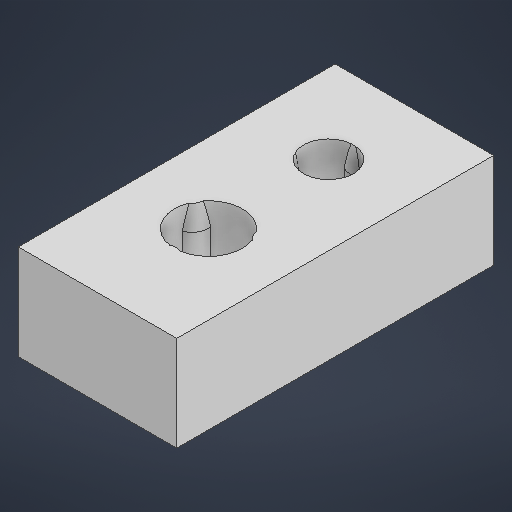
# Autodesk Inventor part: Tolerance_test
Saved by Autodesk Inventor 2025 (Build 290162010, 162A)
## iProperties
Created: 2025-03-10
Part Number: Tolerance_test
Material: Generic
Document SubType Name: Modeling
Designer: tzu98
Density: 1 g/cm^3
Appearance: Default
Author: tzu98
Autodesk Inventor part; units mm, degrees
ref_plane "YZ Plane" through (0, 0, 0) normal (1, 0, 0) x (0, 1, 0)
ref_plane "XZ Plane" through (0, 0, 0) normal (0, 1, 0) x (-1, 0, 0)
ref_plane "XY Plane" through (0, 0, 0) normal (0, 0, 1) x (1, 0, 0)
sketch "Sketch1" plane through (0, 0, 0) normal (0, 0, 1) x (1, 0, 0)
  line L0 (-5, -10) -> (5, -10)
  line L1 (5, -10) -> (5, 10)
  line L2 (5, 10) -> (-5, 10)
  line L3 (-5, 10) -> (-5, -10)
  line L4 (-5, -10) -> (5, 10) construction
  line L5 (5, -10) -> (-5, 10) construction
  circle A0 centre (-10.5904, 5.4479) radius 1.6
  circle A1 centre (-8.5404, 5.4479) radius 0.75
  point P0 (0, 0)
  point P1 (-9.0782, 4.9252)
  point P2 (-9.0782, 5.9707)
  dimension "d0" = 3.2
  dimension "d1" = 2.05
  dimension "d2" = 1.5
  dimension "d29" = 10
  dimension "d30" = 20
  constraints: 12 end point, 2 centre point, 2 midpoint, 2 parallel, 1 horizontal, 1 perpendicular
  measures "d0" diameter of A0
  measures "d1" distance of A1.centre A0.centre
  measures "d2" diameter of A1
  measures "d29" distance between parallel lines of L1 L3
  measures "d30" distance between parallel lines of L2 L0
extrude "Extrusion1" add sketch "Sketch1" along normal blind 6 contours L3 L2 L1 L0
sketch "Sketch2" plane through (0, 0, 6) normal (0, 0, 1) x (1, 0, 0)
  circle A0 centre (0, 4.575) radius 1.575
  line L0 (0, 4.575) -> (0, 6.625)
  circle A1 centre (0, 6.625) radius 0.75
  circle A2 centre (-1.7754, 3.55) radius 0.75
  circle A3 centre (1.7754, 3.55) radius 0.75
  line L1 (0, 0) -> (0, 3)
  circle A4 centre (0, -3) radius 2.15
  line L2 (0, -3) -> (0, -5.8)
  circle A5 centre (0, -5.8) radius 1
  circle A6 centre (2.4249, -1.6) radius 1
  circle A7 centre (-2.4249, -1.6) radius 1
  point P0 (1.0418, 3.3938)
  point P1 (1.5439, 4.2634)
  point P2 (0.5021, 6.0678)
  point P3 (-0.5021, 6.0678)
  point P4 (-1.5439, 4.2634)
  point P5 (-1.0418, 3.3938)
  point P6 (-1.4437, -1.4068)
  point P7 (-2.1016, -2.5463)
  point P8 (-0.6579, -5.0469)
  point P9 (0.6579, -5.0469)
  point P10 (2.1016, -2.5463)
  point P11 (1.4437, -1.4068)
  dimension "d5" = 3.15
  dimension "d6" = 2.05
  dimension "d7" = 1.5
  dimension "d10" = 360
  dimension "d17" = 3
  dimension "d18" = 4.3
  dimension "d19" = 2.8
  dimension "d20" = 2
  dimension "d21" = 3
  dimension "d24" = 360
  constraints: 7 centre point, 6 end point, 4 coincident, 4 vertical, 20 other
  measures "d6" distance of L0.start L0.end
  measures "d7" diameter of A1
  measures "d17" distance of L1.start L1.end
  measures "d18" diameter of A4
  measures "d19" distance of L2.start L2.end
  measures "d20" diameter of A5
  measures "d21" distance of L1.start L2.start
extrude "Extrusion2" cut sketch "Sketch2" against normal blind 10 contours A0 A3 A2 A1 | A4 A5 A7 A6
chamfer "Chamfer1" distance 0.25 angle 80 3 edges at (0, 5.875, 6) (-1.1258, 3.925, 6) (1.1258, 3.925, 6) measured on face at (-4.0339, -0.8488, 6)
chamfer "Chamfer2" distance 0.25 angle 80 3 edges at (-1.5588, -2.1, 6) (1.5588, -2.1, 6) (0, -4.8, 6) measured on face at (-4.0339, -0.8488, 6)
body "Solid1"
